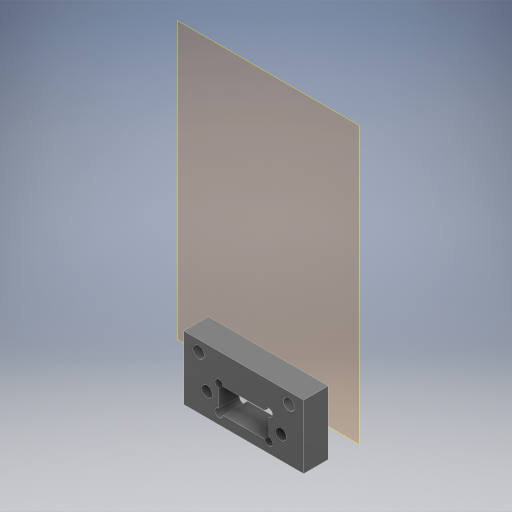
# Autodesk Inventor part: chest connector_fixing part
Saved by Autodesk Inventor 2024 (Build 280153000, 153)
## iProperties
Created: 2024-09-05
Part Number: chest connector_fixing part
Material: PMMA 플라스틱
Document SubType Name: Modeling
Designer: msi
Density: 1.188 g/cm^3
Appearance: 매끄러움 - 검은색
Author: msi
Autodesk Inventor part; units mm, degrees
ref_plane "YZ Plane" through (0, 0, 0) normal (1, 0, 0) x (0, 1, 0)
ref_plane "XZ Plane" through (0, 0, 0) normal (0, 1, 0) x (-1, 0, 0)
ref_plane "XY Plane" through (0, 0, 0) normal (0, 0, 1) x (1, 0, 0)
ref_plane "작업 평면1" through (0, 0, 0) normal (0, 0, 1) x (1, 0, 0)
sketch "스케치1" plane through (0, 0, 0) normal (0, 0, 1) x (1, 0, 0)
  arc A0 (20.1, 4.5766) -> (19.5808, 6.2636) centre (17.1, 4.5766) ccw projected
  line L0 (19.5808, 6.2636) -> (15.5953, 12.1246) projected
  arc A1 (15.5953, 12.1246) -> (13.9414, 13) centre (13.9414, 11) ccw projected
  line L1 (13, 13) -> (13.9414, 13) projected
  arc A2 (14.5, 11.5) -> (13, 13) centre (13, 11.5) ccw projected
  line L2 (14.5, -41.5) -> (14.5, 11.5) projected
  arc A3 (13.5, -42.5) -> (14.5, -41.5) centre (13.5, -41.5) ccw projected
  line L3 (-13.5, -42.5) -> (13.5, -42.5) projected
  arc A4 (-14.5, -41.5) -> (-13.5, -42.5) centre (-13.5, -41.5) ccw projected
  line L4 (-14.5, 11.5) -> (-14.5, -41.5) projected
  arc A5 (-13, 13) -> (-14.5, 11.5) centre (-13, 11.5) ccw projected
  line L5 (-13.9414, 13) -> (-13, 13) projected
  arc A6 (-13.9414, 13) -> (-15.5953, 12.1246) centre (-13.9414, 11) ccw projected
  line L6 (-15.5953, 12.1246) -> (-19.5808, 6.2636) projected
  arc A7 (-19.5808, 6.2636) -> (-20.1, 4.5766) centre (-17.1, 4.5766) ccw projected
  line L7 (-20.1, 4.5766) -> (-20.1, -39.6766) projected
  arc A8 (-20.1, -39.6766) -> (-19.5808, -41.3636) centre (-17.1, -39.6766) ccw projected
  line L8 (-19.5808, -41.3636) -> (-15.8929, -46.7869) projected
  arc A9 (-15.8929, -46.7869) -> (-13.4121, -48.1) centre (-13.4121, -45.1) ccw projected
  line L9 (-13.4121, -48.1) -> (13.4121, -48.1) projected
  arc A10 (13.4121, -48.1) -> (15.8929, -46.7869) centre (13.4121, -45.1) ccw projected
  line L10 (15.8929, -46.7869) -> (19.5808, -41.3636) projected
  arc A11 (19.5808, -41.3636) -> (20.1, -39.6766) centre (17.1, -39.6766) ccw projected
  line L11 (20.1, -39.6766) -> (20.1, 4.5766) projected
  circle A12 centre (-17.3, 4) radius 1.35 projected
  circle A13 centre (-17.3, -18) radius 1.35 projected
  circle A14 centre (-11, -45.3) radius 1.35 projected
  circle A15 centre (17.3, 4) radius 1.35 projected
  circle A16 centre (17.3, -18) radius 1.35 projected
  circle A17 centre (11, -45.3) radius 1.35 projected
  circle A18 centre (-17.3, -40) radius 1.35 projected
  circle A19 centre (17.3, -40) radius 1.35 projected
  arc A20 (-14.6, -41.5) -> (-13.5, -42.6) centre (-13.5, -41.5) ccw
  line L12 (-13.5, -42.6) -> (13.5, -42.6)
  arc A21 (13.5, -42.6) -> (14.6, -41.5) centre (13.5, -41.5) ccw
  line L13 (14.6, -41.5) -> (14.6, 11.5)
  arc A22 (14.6, 11.5) -> (12.2254, 12.9) centre (13, 11.5) ccw
  line L14 (12.2254, 12.9) -> (13.9414, 12.9)
  arc A23 (15.5126, 12.0684) -> (13.9414, 12.9) centre (13.9414, 11) ccw
  line L15 (15.5126, 12.0684) -> (19.4981, 6.2073)
  arc A24 (20, 4.5766) -> (19.4981, 6.2073) centre (17.1, 4.5766) ccw
  line L16 (20, 4.5766) -> (20, -39.6766)
  arc A25 (19.4981, -41.3073) -> (20, -39.6766) centre (17.1, -39.6766) ccw
  line L17 (19.4981, -41.3073) -> (15.8102, -46.7307)
  arc A26 (14.6, -47.7455) -> (15.8102, -46.7307) centre (13.4121, -45.1) ccw
  arc A27 (-15.8102, -46.7307) -> (-14.6, -47.7455) centre (-13.4121, -45.1) ccw
  line L18 (-15.8102, -46.7307) -> (-19.4981, -41.3073)
  arc A28 (-20, -39.6766) -> (-19.4981, -41.3073) centre (-17.1, -39.6766) ccw
  line L19 (-20, -39.6766) -> (-20, 4.5766)
  arc A29 (-19.4981, 6.2073) -> (-20, 4.5766) centre (-17.1, 4.5766) ccw
  line L20 (-19.4981, 6.2073) -> (-15.5126, 12.0684)
  arc A30 (-13.9414, 12.9) -> (-15.5126, 12.0684) centre (-13.9414, 11) ccw
  line L21 (-13.9414, 12.9) -> (-12.2254, 12.9)
  arc A31 (-12.2254, 12.9) -> (-14.6, 11.5) centre (-13, 11.5) ccw
  line L22 (-14.6, 11.5) -> (-14.6, -41.5)
  line L23 (-14.6, -42.6) -> (14.6, -42.6)
  line L24 (14.6, -42.6) -> (14.6, -48.1)
  line L25 (14.6, -48.1) -> (-14.6, -48.1)
  line L26 (-14.6, -48.1) -> (-14.6, -42.6)
  line L27 (-14.6, -48.1) -> (14.6, -48.1)
  line L28 (14.6, -48.1) -> (14.6, -57.1)
  line L29 (14.6, -57.1) -> (-14.6, -57.1)
  line L30 (-14.6, -57.1) -> (-14.6, -48.1)
  circle A32 centre (-11, -45.3) radius 1.4
  circle A33 centre (11, -45.3) radius 1.4
  line L31 (-6.05, -55.65) -> (6.05, -55.65)
  line L32 (6.05, -55.65) -> (6.05, -49.55)
  line L33 (6.05, -49.55) -> (-6.05, -49.55)
  line L34 (-6.05, -49.55) -> (-6.05, -55.65)
  line L35 (-6.05, -55.65) -> (6.05, -49.55) construction
  line L36 (6.05, -55.65) -> (-6.05, -49.55) construction
  line L37 (-14.6, -57.1) -> (14.6, -57.1)
  line L38 (14.6, -57.1) -> (14.6, -58.1)
  line L39 (14.6, -58.1) -> (-14.6, -58.1)
  line L40 (-14.6, -58.1) -> (-14.6, -57.1)
  circle A34 centre (9, -52.6) radius 1.35
  circle A35 centre (-9, -52.6) radius 1.35
  point P0 (0, 0)
  point P1 (0, -52.6)
  point P2 (-13.5, -42.6)
  dimension "d0" = 0.1
  dimension "d1" = 9
  dimension "d2" = 2.8
  dimension "d3" = 2.8
  dimension "d4" = 12.1
  dimension "d5" = 6.1
  dimension "d8" = 1
  dimension "d9" = 2.7
  dimension "d10" = 2.7
  constraints: 58 end point, 24 point on circle, 16 centre point, 8 parallel, 4 horizontal, 4 perpendicular, 2 coincident, 2 midpoint, 2 point on line, 19 other
  measures "d0" distance between parallel lines of L4 L22
  measures "d1" distance of L27.end L28.end
  measures "d2" diameter of A32
  measures "d3" diameter of A33
  measures "d4" distance of L33.end L32.end
  measures "d5" distance of L32.end L31.end
  measures "d8" distance of L37.end L38.end
  measures "d9" diameter of A34
  measures "d10" diameter of A35
extrude "돌출2" add sketch "스케치1" along normal blind 6 contours L24 L25 A10 | A10 L9 A9 L26 L23 L12 L24 | L25 L28 L29 L30 L9 | L25 L26 A9 | L38 L39 L40 L29
sketch "스케치2" plane through (0, 0, 6) normal (0, 0, 1) x (1, 0, 0)
  line L0 (-6.05, -49.55) -> (6.05, -49.55) projected
  line L1 (6.05, -49.55) -> (6.05, -55.65) projected
  line L2 (-6.05, -55.65) -> (-6.05, -49.55) projected
  line L3 (6.05, -55.65) -> (-6.05, -55.65) projected
  circle A0 centre (6.05, -49.55) radius 1
  circle A1 centre (-6.05, -49.55) radius 1
  circle A2 centre (-6.05, -55.65) radius 1
  circle A3 centre (6.05, -55.65) radius 1
  point P0 (0, 0)
  point P1 (5.05, -55.65)
  point P2 (6.05, -54.65)
  dimension "d14" = 2
  dimension "d15" = 2
  dimension "d16" = 2
  dimension "d17" = 2
  constraints: 4 centre point, 4 coincident
  measures "d14" diameter of A0
  measures "d15" diameter of A1
  measures "d16" diameter of A2
  measures "d17" diameter of A3
extrude "돌출3" cut sketch "스케치2" against normal blind 10 contours L2 A1 L0 | L0 A1 L2 | A0 L1 L0 | L0 L1 A0 | A2 L3 L2 | L2 L3 A2 | A3 L3 L1 picked at (5.393, -55.7298)
